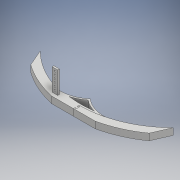
# Autodesk Inventor part: Kick male
Saved by Autodesk Inventor 2018 (Build 220112000, 112)
## iProperties
Created: 2019-11-10
Part Number: Kick male
Material: Типовые
Document SubType Name: Modeling
Designer: cosko
Density: 1 g/cm^3
Appearance: По умолчанию
Author: cosko
Autodesk Inventor part; units mm, degrees
ref_plane "YZ Plane" through (0, 0, 0) normal (1, 0, 0) x (0, 1, 0)
ref_plane "XZ Plane" through (0, 0, 0) normal (0, 1, 0) x (-1, 0, 0)
ref_plane "XY Plane" through (0, 0, 0) normal (0, 0, 1) x (1, 0, 0)
sketch "Эскиз1" plane through (0, 0, 0) normal (0, 0, 1) x (1, 0, 0)
  line L0 (39.103634, -30) -> (-39.103634, -30)
  line L1 (-120, 30) -> (120, -30) construction
  line L2 (120, 30) -> (-120, -30) construction
  line L3 (0, -30) -> (0, -27) construction
  arc A0 (-120, 30) -> (120, 30) centre (0, 150.415946) ccw
  arc A1 (-107.0236, 0) -> (-39.103634, -30) centre (0, 150.415946) ccw
  arc A2 (39.103634, -30) -> (107.0236, 0) centre (0, 150.415946) ccw
  line L4 (120, 30) -> (107.0236, 0)
  line L5 (-120, 30) -> (-107.0236, 0)
  point P0 (0, 0)
  dimension "d0" = 240
  dimension "d1" = 60
  dimension "d6" = 3
  dimension "d7" = 170
  constraints: 12 end point, 6 point on circle, 3 centre point, 3 midpoint, 1 vertical
  measures "d0" distance of L1.end L2.end
  measures "d1" distance of L2.start L1.end
  measures "d6" distance of L3.start L3.end
  measures "d7" radius of A0
extrude "Выдавливание1" add sketch "Эскиз1" along normal blind 12
sketch "Эскиз2" plane through (0, 0, 12) normal (0, 0, 1) x (1, 0, 0)
  line L0 (-39.103634, -30) -> (39.103634, -30)
  line L1 (-39.103634, -30) -> (39.103634, -30) construction
  line L2 (0, -30) -> (10, -30) construction
  line L3 (0, -30) -> (-10, -30) construction
  arc A0 (-120, 30) -> (120, 30) centre (0, 150.415946) ccw
  line L4 (-120, 30) -> (-107.0236, 0)
  arc A1 (-107.0236, 0) -> (-39.103634, -30) centre (0, 150.415946) ccw
  arc A2 (39.103634, -30) -> (107.0236, 0) centre (0, 150.415946) ccw
  line L5 (107.0236, 0) -> (120, 30)
  point P0 (0, 0)
  point P1 (-12, -3)
  point P2 (12, -3)
  dimension "d4" = 10
  dimension "d5" = 10
  constraints: 4 end point, 4 other
  measures "d4" distance of L2.start L2.end
  measures "d5" distance of L2.start L3.end
sketch "Эскиз3" plane through (0, 0, 12) normal (0, 0, 1) x (1, 0, 0)
  line L0 (-39.103634, -30) -> (39.103634, -30) construction
  line L1 (0, -30) -> (0, -19.584054) construction
  arc A0 (-120, 30) -> (120, 30) centre (0, 150.415946) ccw construction
  line L2 (0, -24.792027) -> (-58.147862, -24.792027) construction
  arc A1 (-107.0236, 0) -> (-39.103634, -30) centre (0, 150.415946) ccw construction
  arc A2 (39.103634, -30) -> (107.0236, 0) centre (0, 150.415946) ccw construction
  line L3 (58.147862, -24.792027) -> (0, -24.792027) construction
  line L4 (0, -24.792027) -> (0, -27.792027)
  line L5 (0, -27.792027) -> (0, -21.792027)
  line L6 (0, -24.792027) -> (6, -24.792027) construction
  line L7 (0, -26.524078) -> (3, -28.256129)
  line L8 (0, -24.792027) -> (6.928203, -24.792027) construction
  line L9 (3, -28.256129) -> (3, -24.792027)
  line L10 (0, -23.059976) -> (3, -21.327925)
  line L11 (0, -24.792027) -> (6.928203, -24.792027) construction
  line L12 (3, -21.327925) -> (3, -24.792027)
  line L13 (0, -24.792027) -> (-3, -24.792027) construction
  line L14 (0, -23.059976) -> (0, -19.584054)
  line L15 (0, -26.524078) -> (0, -30)
  point P0 (0, 0)
  dimension "d8" = 3
  dimension "d9" = 6
  dimension "d10" = 6
  dimension "d11" = 30
  dimension "d12" = 30
  dimension "d13" = 3
  constraints: 30 end point, 6 point on line, 3 horizontal, 3 point on circle, 3 vertical, 2 collinear, 1 midpoint, 1 perpendicular
  measures "d8" distance of L4.start L4.end
  measures "d9" distance of L4.end L5.end
  measures "d10" distance of L6.start L6.end
  measures "d11" angle of L7 L8
  measures "d12" angle of L11 L10
  measures "d13" distance of L13.start L13.end
sketch "Эскиз4" plane through (0, 0, 0) normal (0, 0, -1) x (-1, 0, 0)
  line L0 (-3, -28.256129) -> (-3, -24.792027)
  line L1 (0, -26.524078) -> (-3, -28.256129)
  line L2 (-3, -21.327925) -> (-3, -24.792027)
  line L3 (0, -23.059976) -> (-3, -21.327925)
  line L4 (0, -24.792027) -> (0, -27.792027)
  line L5 (0, -27.792027) -> (0, -21.792027)
  point P0 (0, 0)
ref_plane "РабПлоскость1" through (3, -21.327925, 12) normal (0.5, -0.8660254, 0) x (-0.8660254, -0.5, 0)
ref_plane "РабПлоскость2" through (3, -21.327925, 0) normal (-1, 0, 0) x (0, -1, 0)
ref_plane "РабПлоскость3" through (0, -26.524078, 12) normal (0.5, 0.8660254, 0) x (0.8660254, -0.5, 0)
ref_plane "РабПлоскость4" through (0, -19.584054, 12) normal (1, 0, 0) x (0, -1, 0)
ref_plane "РабПлоскость5" through (0, -26.524078, 0) normal (-1, 0, 0) x (0, -1, 0)
split body "Разделение1" sketch "Эскиз3" result two bodies curves L15 L7 L9 L12 L10 L14 first body at (-18.576653, -26.256352, 0.5)
sketch "Эскиз5" plane through (0, 0, 12) normal (0, 0, 1) x (1, 0, 0)
  line L0 (0, -19.584054) -> (0, -23.059976)
  arc A0 (-120, 30) -> (0, -19.584054) centre (0, 150.415946) ccw
  line L1 (-120, 30) -> (-107.0236, 0)
  arc A1 (-107.0236, 0) -> (-39.103634, -30) centre (0, 150.415946) ccw
  line L2 (-39.103634, -30) -> (0, -30)
  line L3 (0, -26.524078) -> (0, -30)
  line L4 (3, -28.256129) -> (0, -26.524078)
  line L5 (3, -21.327925) -> (3, -28.256129)
  line L6 (0, -23.059976) -> (3, -21.327925)
  line L7 (39.103634, -30) -> (0, -30)
  line L8 (0, -19.584054) -> (0, -23.059976)
  line L9 (0, -23.059976) -> (3, -21.327925)
  line L10 (3, -21.327925) -> (3, -28.256129)
  line L11 (3, -28.256129) -> (0, -26.524078)
  line L12 (0, -26.524078) -> (0, -30)
  line L13 (0, -30) -> (39.103634, -30)
  arc A2 (39.103634, -30) -> (107.0236, 0) centre (0, 150.415946) ccw
  line L14 (107.0236, 0) -> (120, 30)
  arc A3 (0, -19.584054) -> (120, 30) centre (0, 150.415946) ccw
  arc A4 (0, -19.584054) -> (120, 30) centre (0, 150.415946) ccw construction
  line L15 (0, -19.584054) -> (0, 0.415946) construction
  arc A5 (0, -19.584054) -> (120, 30) centre (0, 150.415946) ccw
  arc A6 (0, 0.415946) -> (41.962718, -14.323637) centre (39.482655, 45.718245) ccw
  arc A7 (-41.962718, -14.323637) -> (0, 0.415946) centre (-39.482655, 45.718245) ccw
  arc A8 (-41.962718, -14.323637) -> (41.962718, -14.323637) centre (0, 150.415946) ccw
  arc A9 (0, -3.494119) -> (22.536422, -15.056438) centre (39.482655, 45.718245) ccw
  arc A10 (-22.536422, -15.056438) -> (22.536422, -15.056438) centre (0, 150.415946) ccw
  arc A11 (-22.536422, -15.056438) -> (0, -3.494119) centre (-39.482655, 45.718245) ccw
  point P0 (0, 0)
  dimension "d15" = 20
  dimension "d18" = 3
  constraints: 13 point on circle, 6 centre point, 2 end point, 2 symmetric about line, 1 vertical, 3 other
  measures "d15" distance of L0.start L15.end
  measures "d18" radial gap between concentric circles of A7 A11
extrude "Выдавливание2" add sketch "Эскиз5" against normal up to surface (12 mm away) contours A0 A7 A6 A3 bodies 2
sketch "Эскиз6" plane through (0, 0, 12) normal (0, 0, 1) x (1, 0, 0)
  arc A0 (-22.536422, -15.056438) -> (0, -3.494119) centre (-39.482655, 45.718245) ccw construction
  arc A1 (0, -3.494119) -> (22.536422, -15.056438) centre (39.482655, 45.718245) ccw construction
  arc A2 (-22.536422, -15.056438) -> (22.536422, -15.056438) centre (0, 150.415946) ccw construction
  line L0 (0, -19.584054) -> (0, -23.059976) construction
  arc A3 (0, -19.584054) -> (41.962718, -14.323637) centre (0, 150.415946) ccw construction
  arc A4 (0, 0.415946) -> (41.962718, -14.323637) centre (39.482655, 45.718245) ccw construction
  arc A5 (-41.962718, -14.323637) -> (0, 0.415946) centre (-39.482655, 45.718245) ccw construction
  arc A6 (-120, 30) -> (-41.962718, -14.323637) centre (0, 150.415946) ccw construction
  line L1 (-120, 30) -> (-107.0236, 0) construction
  arc A7 (-107.0236, 0) -> (-39.103634, -30) centre (0, 150.415946) ccw construction
  line L2 (-39.103634, -30) -> (0, -30) construction
  line L3 (0, -26.524078) -> (0, -30) construction
  line L4 (3, -28.256129) -> (0, -26.524078) construction
  line L5 (3, -21.327925) -> (3, -28.256129) construction
  line L6 (0, -23.059976) -> (3, -21.327925) construction
  line L7 (0, -19.584054) -> (0, -23.059976) construction
  line L8 (0, -23.059976) -> (3, -21.327925) construction
  line L9 (3, -21.327925) -> (3, -28.256129) construction
  line L10 (3, -28.256129) -> (0, -26.524078) construction
  line L11 (0, -26.524078) -> (0, -30) construction
  line L12 (0, -30) -> (39.103634, -30) construction
  arc A8 (39.103634, -30) -> (107.0236, 0) centre (0, 150.415946) ccw construction
  line L13 (107.0236, 0) -> (120, 30) construction
  arc A9 (0, -19.584054) -> (120, 30) centre (0, 150.415946) ccw construction
  line L14 (107.0236, 0) -> (-107.0236, 0) construction
  line L15 (0, -30) -> (-100, -30) construction
  line L16 (0, -30) -> (100, -30) construction
  line L17 (100, -30) -> (-34.663, -30) construction
  line L18 (-100, -30) -> (-44.663, -30) construction
  line L19 (-34.663, -30) -> (-44.663, -30) construction
  line L20 (-34.663, -31.5) -> (-44.663, -31.5) construction
  line L21 (-44.663, -31.5) -> (-44.663, -28.5) construction
  line L22 (-44.663, -28.5) -> (-34.663, -28.5) construction
  line L23 (-34.663, -28.5) -> (-34.663, -31.5) construction
  line L24 (-34.663, -31.5) -> (-44.663, -28.5) construction
  line L25 (-44.663, -31.5) -> (-34.663, -28.5) construction
  line L26 (-34.663, -30) -> (-34.663, -14.323637) construction
  line L27 (-44.663, -30) -> (-44.663, -13.612151) construction
  line L28 (-34.663, -22.161819) -> (-44.663, -22.161819) construction
  line L29 (-34.663, -20.661819) -> (-44.663, -20.661819)
  line L30 (-44.663, -20.661819) -> (-44.663, -23.661819)
  line L31 (-44.663, -23.661819) -> (-34.663, -23.661819)
  line L32 (-34.663, -23.661819) -> (-34.663, -20.661819)
  line L33 (-34.663, -20.661819) -> (-44.663, -23.661819) construction
  line L34 (-44.663, -20.661819) -> (-34.663, -23.661819) construction
  point P0 (0, 0)
  point P1 (-39.663, -30)
  point P2 (-39.663, -22.161819)
  dimension "d19" = 100
  dimension "d20" = 100
  dimension "d21" = 134.663
  dimension "d22" = 55.337
  dimension "d23" = 3
  dimension "d24" = 3
  constraints: 42 end point, 7 midpoint, 6 point on line, 4 parallel, 3 horizontal, 3 perpendicular, 2 vertical, 1 collinear, 1 point on circle
  measures "d19" distance of L11.end L15.end
  measures "d20" distance of L2.end L16.end
  measures "d21" distance of L16.end L17.end
  measures "d22" distance of L15.end L18.end
  measures "d23" distance of L20.end L21.end
  measures "d24" distance of L30.end L29.end
extrude "Выдавливание3" add sketch "Эскиз6" along normal blind 40 bodies 2
sketch "Эскиз7" plane through (-44.663, -20.661819, 12) normal (0, 1, 0) x (1, 0, 0)
  line L0 (0, 0) -> (10, 0) projected
  line L1 (0, 0) -> (0, -40) projected
  line L2 (10, -40) -> (0, -40) projected
  line L3 (10, 0) -> (10, -40) projected
  line L4 (0, 0) -> (0, -5.5) construction
  line L5 (0, 0) -> (0, -40) construction
  line L6 (0, -5.5) -> (10, -5.5) construction
  line L7 (5, -40) -> (5, 0) construction
  line L8 (0, 0) -> (10, 0) construction
  circle A0 centre (5, -5.5) radius 1.5
  line L9 (5, -5.5) -> (5, -11.5) construction
  circle A1 centre (5, -11.5) radius 1.5
  circle A2 centre (5, -17.5) radius 1.5
  circle A3 centre (5, -23.5) radius 1.5
  circle A4 centre (5, -29.5) radius 1.5
  circle A5 centre (5, -35.5) radius 1.5
  point P0 (44.663, 12)
  dimension "d27" = 5.5
  dimension "d28" = 3
  dimension "d29" = 6
  dimension "d30" = 3
  dimension "d38" = 6
  dimension "d45" = 6
  constraints: 8 end point, 6 centre point, 4 point on line, 3 midpoint, 2 vertical, 1 coincident, 1 perpendicular, 8 other
  measures "d27" distance of L0.start L4.end
  measures "d28" diameter of A0
  measures "d29" distance of L9.start L9.end
  measures "d30" diameter of A1
  measures "d38" distance of A1.centre A2.centre
  measures "d45" distance of A3.centre A4.centre
extrude "Выдавливание4" cut sketch "Эскиз7" against normal blind 6 contours A0 | A1 | A2 | A3 | A4 | A5 bodies 2
equation "\"d31\" = d38"
